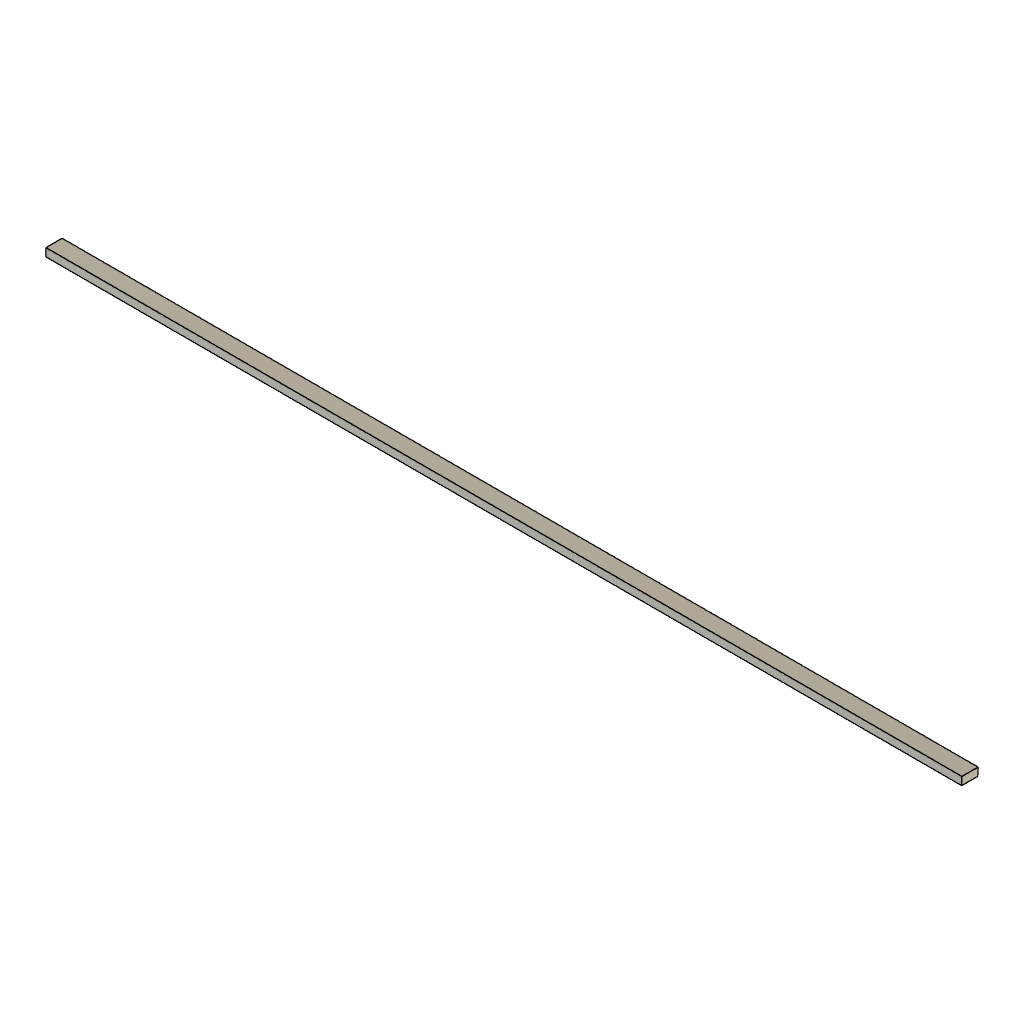
A3 (Autodesk Fusion 360 design; units mm, degrees)
part number: 2026-09-08-20-25-06-183
Autodesk Fusion 360 part; units mm, degrees
sketch "Sketch1" plane through (0, 0, 0) normal (0, 1, 0) x (1, 0, 0)
  line L0 (0, 0) -> (0, -6.35)
  line L1 (0, -6.35) -> (713.8821, -6.35)
  line L2 (0, 0) -> (713.7399, 0)
  line L3 (713.7399, 0) -> (713.8821, -6.35)
  dimension "d1" = 6.35
  dimension "d2" = 713.8821
  constraint coincident L0.start L2.start
  constraint vertical L0
  constraint perpendicular L0 L1
  constraint perpendicular L0 L2
  measures "d1" distance of L0.start L0.end
  measures "d2" distance of L0.end L1.end
extrude "Extrude2" add sketch "Sketch1" along normal blind 12.7
equation "d1 = Height"
equation "d2 = Length"
equation "Width = 0.500 in"
equation "Height = 0.250 in"
equation "Load = 400.00 lbforce"
equation "Elastic_Modulus = 9993100 psi"
equation "Max_Delta = 0.009 in"
equation "Length = Width * Height * Max_Delta * Elastic_Modulus / Load"
equation "d11 = Width"
